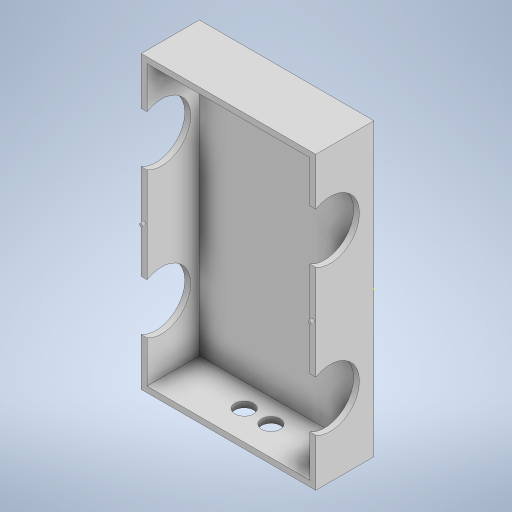
# Autodesk Inventor part: broomba top
Saved by Autodesk Inventor 2023.2 (Build 272271000, 271)
## iProperties
Created: 2023-07-21
Part Number: broomba top
Material: Generic
Document SubType Name: Modeling
Designer: 30067459
Density: 1 g/cm^3
Appearance: Default
Author: 30067459
Autodesk Inventor part; units mm, degrees
ref_plane "YZ Plane" through (0, 0, 0) normal (1, 0, 0) x (0, 1, 0)
ref_plane "XZ Plane" through (0, 0, 0) normal (0, 1, 0) x (-1, 0, 0)
ref_plane "XY Plane" through (0, 0, 0) normal (0, 0, 1) x (1, 0, 0)
sketch "Sketch1" plane through (0, 0, 0) normal (0, 0, 1) x (1, 0, 0)
  line L0 (-75, 125) -> (75, 125)
  line L1 (75, 125) -> (75, -125)
  line L2 (75, -125) -> (-75, -125)
  line L3 (-75, -125) -> (-75, 125)
  line L4 (-75, 125) -> (75, -125) construction
  line L5 (75, 125) -> (-75, -125) construction
  point P0 (0, 0)
  dimension "d0" = 150
  dimension "d1" = 250
  constraints: 12 end point, 2 midpoint, 2 parallel, 1 horizontal, 1 perpendicular
  measures "d0" distance of L1.end L2.end
  measures "d1" distance of L0.end L1.end
extrude "Extrusion1" add sketch "Sketch1" along normal blind 50
shell "Shell1" thickness 5 removed faces 1 at (-25, -41.6667, 50)
sketch "Sketch2" plane through (-75, -125, 0) normal (0, -1, 0) x (1, 0, 0)
  line L0 (75, 0) -> (75, 50)
  line L1 (150, 50) -> (0, 50) projected
  line L2 (52.5, 35) -> (97.5, 35)
  line L3 (97.5, 35) -> (97.5, 15)
  line L4 (97.5, 15) -> (52.5, 15)
  line L5 (52.5, 15) -> (52.5, 35)
  line L6 (52.5, 35) -> (97.5, 15) construction
  line L7 (97.5, 35) -> (52.5, 15) construction
  line L8 (97.5, 25) -> (94.5, 25)
  line L9 (94.5, 25) -> (78.5, 25)
  line L10 (52.5, 25) -> (55.5, 25)
  line L11 (55.5, 25) -> (71.5, 25)
  circle A0 centre (86.5, 25) radius 8
  circle A1 centre (63.5, 25) radius 8
  point P0 (75, 25)
  dimension "d5" = 45
  dimension "d6" = 20
  dimension "d7" = 3
  dimension "d8" = 16
  dimension "d9" = 3
  dimension "d10" = 16
  dimension "d11" = 16
  dimension "d12" = 16
  constraints: 22 end point, 8 midpoint, 3 horizontal, 2 centre point, 2 parallel, 2 point on line, 1 perpendicular
  measures "d5" distance of L3.end L4.end
  measures "d6" distance of L2.end L3.end
  measures "d7" distance of L8.start L8.end
  measures "d8" distance of L8.end L9.end
  measures "d9" distance of L10.start L10.end
  measures "d10" distance of L10.end L11.end
  measures "d11" diameter of A0
  measures "d12" diameter of A1
extrude "Extrusion2" cut sketch "Sketch2" against normal blind 86 contours A1 L11 | L11 A1 | A0 L9 | L9 A0
sketch "Sketch3" plane through (-75, -125, 0) normal (-1, 0, 0) x (0, 0, 1)
  line L0 (0, 125) -> (50, 125)
  line L1 (50, 5) -> (50, 245) projected
  line L2 (25, 125) -> (25, 0)
  line L3 (0, 0) -> (50, 0) projected
  line L4 (25, 62.5) -> (50, 62.5)
  circle A0 centre (37.5, 62.5) radius 25
  dimension "d15" = 50
  constraints: 6 end point, 5 midpoint, 1 centre point, 1 perpendicular, 1 point on line
  measures "d15" diameter of A0
extrude "Extrusion3" cut sketch "Sketch3" against normal blind 192.25 contours A0 L1 L4 L2 | L2 A0 | A0 L1 | L4 L1 A0 L2
sketch "Sketch4" plane through (-75, -125, 0) normal (-1, 0, 0) x (0, 0, 1)
  line L0 (0, 125) -> (50, 125)
  line L1 (50, 245) -> (50, 84.1506) projected
  line L2 (25, 125) -> (25, 250)
  line L3 (0, 250) -> (50, 250) projected
  line L4 (25, 187.5) -> (50, 187.5)
  circle A0 centre (37.5, 187.5) radius 25
  dimension "d18" = 50
  constraints: 6 end point, 4 midpoint, 2 horizontal, 1 centre point, 1 point on line
  measures "d18" diameter of A0
extrude "Extrusion4" cut sketch "Sketch4" against normal blind 216.5 contours A0 L2 | L2 L4 L1 A0 | L1 A0 | L2 A0 L1 L4
sketch "Sketch5" plane through (0, 0, 50) normal (0, 0, 1) x (1, 0, 0)
  line L0 (-75, 40.8494) -> (-75, -40.8494) projected
  line L1 (-75, 0) -> (-70, 0)
  line L2 (-70, -40.8494) -> (-70, 40.8494) projected
  circle A0 centre (-72.5, 0) radius 1.25
  point P0 (0, 0)
  dimension "d21" = 2.5
  constraints: 3 midpoint, 2 end point, 1 centre point
  measures "d21" diameter of A0
extrude "Extrusion5" add sketch "Sketch5" along normal blind 2.75
sketch "Sketch6" plane through (0, 0, 50) normal (0, 0, 1) x (1, 0, 0)
  line L0 (70, 40.8494) -> (70, -40.8494) projected
  line L1 (70, 0) -> (75, 0)
  line L2 (75, -125) -> (75, 125) projected
  circle A0 centre (72.5, 0) radius 1.25
  point P0 (0, 0)
  dimension "d24" = 2.5
  constraints: 3 midpoint, 2 end point, 1 centre point
  measures "d24" diameter of A0
extrude "Extrusion6" add sketch "Sketch6" along normal blind 2.75
sketch "Sketch7" plane through (75, -125, 0) normal (1, 0, 0) x (0, 0, -1)
  point P0 (0, 125)
body "Solid1"
